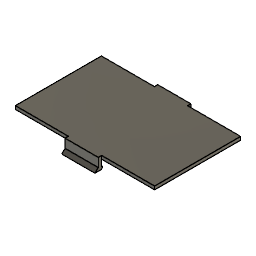
Tapa Pilas (Autodesk Fusion 360 design; units mm, degrees)
part number: 2026-08-17-13-49-44-268
Autodesk Fusion 360 part; units mm, degrees
sketch "Boceto1" plane through (0, 0, 0) normal (0, 0, 1) x (1, 0, 0)
  line L0 (41.9, 25.9) -> (-41.9, 25.9)
  line L1 (-41.9, 25.9) -> (-41.9, -25.9)
  line L2 (-41.9, -25.9) -> (41.9, -25.9)
  line L3 (41.9, -25.9) -> (41.9, 25.9)
  line L4 (41.9, 25.9) -> (-41.9, -25.9) construction
  line L5 (-41.9, 25.9) -> (41.9, -25.9) construction
  dimension "d1" = 83.8
  dimension "d2" = 51.8
  constraint horizontal L0
  constraint perpendicular L0 L1
  constraint parallel L0 L2
  constraint parallel L1 L3
  constraint coincident L4 origin
  constraint coincident L5 origin
  measures "d1" distance of L1.end L2.end
  measures "d2" distance of L0.end L1.end
extrude "Extruir1" add sketch "Boceto1" along normal blind 2
sketch "Boceto4" plane through (0, 0, 0) normal (1, 0, 0) x (0, 1, 0)
  line L0 (25.9, 2) -> (27.9, 2)
  line L1 (27.9, 2) -> (27.9, -5.3)
  line L2 (27.9, -5.3) -> (25.9, -5.3)
  line L3 (25.9, -5.3) -> (25.9, 2)
  line L4 (25.9, -5.3) -> (24.8996, -3.8)
  line L5 (25.9, -5.3) -> (27.703, -5.3) construction
  line L6 (24.8996, -3.8) -> (25.9, -3.8)
  line L7 (27.9, -5.3) -> (29.9, -5.3)
  line L8 (27.9, -5.3) -> (27.9, -3.3)
  line L9 (27.9, -3.3) -> (29.9, -5.3)
  line L10 (0, 7.5) -> (0, -4)
  line L11 (-25.9, -5.3) -> (-25.9, 2)
  line L12 (-25.9, 2) -> (-27.9, 2)
  line L13 (-27.9, 2) -> (-27.9, -5.3)
  line L14 (-27.9, -5.3) -> (-29.9, -5.3)
  line L15 (-27.9, -5.3) -> (-27.9, -3.3)
  line L16 (-27.9, -3.3) -> (-29.9, -5.3)
  line L17 (-24.8996, -3.8) -> (-25.9, -3.8)
  line L18 (-25.9, -5.3) -> (-24.8996, -3.8)
  line L19 (-25.9, -5.3) -> (-27.703, -5.3) construction
  line L20 (-27.9, -5.3) -> (-25.9, -5.3)
  dimension "d20" = 2
  dimension "d21" = 7.3
  dimension "d29" = 1.0004
  dimension "d30" = 1.803
  dimension "d31" = 2
  dimension "d32" = 2
  constraint horizontal L0
  constraint vertical L1
  constraint horizontal L2
  constraint vertical L3
  constraint horizontal L5
  constraint coincident L3 L6.end
  constraint perpendicular L3 L6
  constraint perpendicular L1 L7
  constraint perpendicular L7 L8
  constraint vertical L10
  constraint symmetric L0.start L10 L11.end
  constraint symmetric L0.end L10 L12.end
  constraint symmetric L1.end L10 L13.end
  constraint symmetric L2.end L10 L11.start
  constraint symmetric L4.end L10 L17.start
  constraint symmetric L5.end L10 L19.end
  constraint symmetric L6.end L10 L17.end
  constraint symmetric L7.end L10 L14.end
  constraint symmetric L8.end L10 L15.end
  measures "d20" distance of L0.start L0.end
  measures "d21" distance of L0.start L2.end
  measures "d29" distance of L4.end L6.end
  measures "d30" distance of L2.end L4.end
  measures "d31" distance of L1.end L7.end
  measures "d32" distance of L1.end L8.end
extrude "Extruir5" add sketch "Boceto4" along normal mid plane 20
fillet "Empalme1" radius 0.25 2 edges at (0, 24.8996, -3.8) (0, -24.8996, -3.8)
equation "d21 = 2 mm + 5.3 mm"
